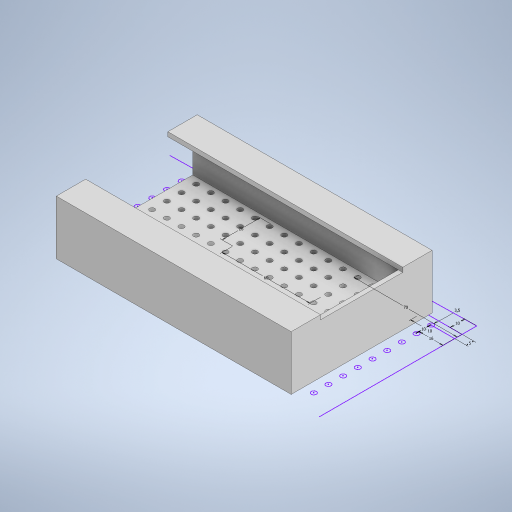
# Autodesk Inventor part: support batterie
Saved by Autodesk Inventor 2024 (Build 280153000, 153)
## iProperties
Created: 2024-02-10
Part Number: support batterie
Material: Generic
Document SubType Name: Modeling
Designer: Pooo
Density: 1 g/cm^3
Appearance: Default
Author: Pooo
## iProperties of the stored document support batterie_3DPrint.ipt
Created: 2024-02-22
Part Number: support batterie_3DPrint
Material: Generic
Document SubType Name: Modeling
Designer: Pooo
Density: 1 g/cm^3
Appearance: Default
Author: Pooo
Autodesk Inventor part; units mm, degrees
ref_plane "YZ Plane" through (0, 0, 0) normal (1, 0, 0) x (0, 1, 0)
ref_plane "XZ Plane" through (0, 0, 0) normal (0, 1, 0) x (-1, 0, 0)
ref_plane "XY Plane" through (0, 0, 0) normal (0, 0, 1) x (1, 0, 0)
sketch "Sketch1" plane through (0, 0, 0) normal (0, 1, 0) x (-1, 0, 0)
  point P0 (0, 0)
sketch "Sketch2" plane through (0, 0, 0) normal (0, 1, 0) x (-1, 0, 0)
  line L0 (43.1586, 43.7586) -> (-113.8414, 43.7586)
  line L1 (-113.8414, 43.7586) -> (-113.8414, -46.2414)
  line L2 (-113.8414, -46.2414) -> (43.1586, -46.2414)
  line L3 (43.1586, -46.2414) -> (43.1586, 43.7586)
  line L4 (43.1586, -46.2414) -> (-113.8414, -46.2414)
  line L5 (-113.8414, -46.2414) -> (-113.8414, -49.2414)
  line L6 (-113.8414, -49.2414) -> (43.1586, -49.2414)
  line L7 (43.1586, -49.2414) -> (43.1586, -46.2414)
  line L8 (43.1586, 43.7586) -> (-113.8414, 43.7586)
  line L9 (-113.8414, 43.7586) -> (-113.8414, 46.7586)
  line L10 (-113.8414, 46.7586) -> (43.1586, 46.7586)
  line L11 (43.1586, 46.7586) -> (43.1586, 43.7586)
  line L12 (-113.8414, 46.7586) -> (-116.8414, 46.7586)
  line L13 (-116.8414, 46.7586) -> (-116.8414, -49.2414)
  line L14 (-116.8414, -49.2414) -> (-113.8414, -49.2414)
  line L15 (-113.8414, -49.2414) -> (-113.8414, 46.7586)
  point P0 (0, 0)
  dimension "d0" = 90
  dimension "d1" = 157
  dimension "d2" = 3
  dimension "d3" = 3
  dimension "d4" = 3
  constraints: 32 end point, 8 parallel, 4 horizontal, 4 perpendicular
  measures "d0" distance of L2.end L0.start
  measures "d1" distance of L1.end L2.end
  measures "d2" distance of L4.end L5.end
  measures "d3" distance of L8.end L9.end
  measures "d4" distance of L14.end L13.end
extrude "Extrusion1" add sketch "Sketch2" along normal blind 3
sketch "Sketch3" plane through (0, 3, 0) normal (0, 1, 0) x (1, 0, 0)
  line L0 (-43.1586, -46.7586) -> (116.8414, -46.7586) projected
  line L1 (116.8414, -46.7586) -> (116.8414, 49.2414) projected
  line L2 (-43.1586, -46.7586) -> (116.8414, -46.7586)
  line L3 (116.8414, -46.7586) -> (116.8414, -43.7586)
  line L4 (116.8414, -43.7586) -> (-43.1586, -43.7586)
  line L5 (-43.1586, -43.7586) -> (-43.1586, -46.7586)
  line L6 (116.8414, 49.2414) -> (-43.1586, 49.2414) projected
  line L7 (-43.1586, 49.2414) -> (116.8414, 49.2414)
  line L8 (116.8414, 49.2414) -> (116.8414, 46.2414)
  line L9 (116.8414, 46.2414) -> (-43.1586, 46.2414)
  line L10 (-43.1586, 46.2414) -> (-43.1586, 49.2414)
  line L11 (116.8414, -43.7586) -> (113.8414, -43.7586)
  line L12 (113.8414, -43.7586) -> (113.8414, 46.2414)
  line L13 (113.8414, 46.2414) -> (116.8414, 46.2414)
  line L14 (116.8414, 46.2414) -> (116.8414, -43.7586)
  point P0 (0, 0)
  dimension "d7" = 3
  dimension "d8" = 3
  dimension "d9" = 3
  constraints: 24 end point, 6 parallel, 3 horizontal, 3 perpendicular, 3 point on line
  measures "d7" distance of L3.end L2.end
  measures "d8" distance of L7.end L8.end
  measures "d9" distance of L12.end L13.end
extrude "Extrusion3" add sketch "Sketch3" along normal blind 31
sketch "Sketch8" plane through (0, 34, 0) normal (0, 1, 0) x (1, 0, 0)
  line L0 (116.8414, -46.7586) -> (116.8414, 49.2414) projected
  line L1 (-43.1586, 49.2414) -> (116.8414, 49.2414)
  line L2 (116.8414, 49.2414) -> (116.8414, 29.2414)
  line L3 (116.8414, 29.2414) -> (-43.1586, 29.2414)
  line L4 (-43.1586, 29.2414) -> (-43.1586, 49.2414)
  line L5 (116.8414, -46.7586) -> (-43.1586, -46.7586)
  line L6 (-43.1586, -46.7586) -> (-43.1586, -26.7586)
  line L7 (-43.1586, -26.7586) -> (116.8414, -26.7586)
  line L8 (116.8414, -26.7586) -> (116.8414, -46.7586)
  point P0 (0, 0)
  dimension "d23" = 20
  dimension "d24" = 20
  constraints: 16 end point, 4 parallel, 2 horizontal, 2 perpendicular, 2 point on line
  measures "d23" distance of L1.end L2.end
  measures "d24" distance of L5.end L6.end
extrude "Extrusion4" add sketch "Sketch8" along normal blind 3
sketch "Sketch12" plane through (-65.6586, 0, -52.9186) normal (0, -1, 0) x (0, 0, -1)
  line L0 (0, 0) -> (3.9725, 205.1618)
  line L1 (3.9725, 205.1618) -> (-6.0275, 205.1618)
  line L2 (-103.3545, 205.1618) -> (3.9725, 205.1618)
  line L3 (-6.0275, 205.1618) -> (-11.0275, 205.1618)
  line L4 (-11.0275, 205.1618) -> (-11.0275, 189.1618)
  circle A0 centre (-11.0275, 189.1618) radius 1.75
  circle A1 centre (-11.0275, 179.1618) radius 1.75
  circle A2 centre (-11.0275, 169.1618) radius 1.75
  circle A3 centre (-11.0275, 159.1618) radius 1.75
  circle A4 centre (-11.0275, 149.1618) radius 1.75
  circle A5 centre (-11.0275, 139.1618) radius 1.75
  circle A6 centre (-11.0275, 129.1618) radius 1.75
  circle A7 centre (-11.0275, 119.1618) radius 1.75
  circle A8 centre (-11.0275, 109.1618) radius 1.75
  circle A9 centre (-11.0275, 99.1618) radius 1.75
  circle A10 centre (-11.0275, 89.1618) radius 1.75
  circle A11 centre (-11.0275, 79.1618) radius 1.75
  circle A12 centre (-11.0275, 69.1618) radius 1.75
  circle A13 centre (-11.0275, 59.1618) radius 1.75
  circle A14 centre (-11.0275, 49.1618) radius 1.75
  circle A15 centre (-11.0275, 39.1618) radius 1.75
  circle A16 centre (-11.0275, 29.1618) radius 1.75
  circle A17 centre (-11.0275, 19.1618) radius 1.75
  circle A18 centre (-21.0275, 189.1618) radius 1.75
  circle A19 centre (-21.0275, 179.1618) radius 1.75
  circle A20 centre (-21.0275, 169.1618) radius 1.75
  circle A21 centre (-21.0275, 159.1618) radius 1.75
  circle A22 centre (-21.0275, 149.1618) radius 1.75
  circle A23 centre (-21.0275, 139.1618) radius 1.75
  circle A24 centre (-21.0275, 129.1618) radius 1.75
  circle A25 centre (-21.0275, 119.1618) radius 1.75
  circle A26 centre (-21.0275, 109.1618) radius 1.75
  circle A27 centre (-21.0275, 99.1618) radius 1.75
  circle A28 centre (-21.0275, 89.1618) radius 1.75
  circle A29 centre (-21.0275, 79.1618) radius 1.75
  circle A30 centre (-21.0275, 69.1618) radius 1.75
  circle A31 centre (-21.0275, 59.1618) radius 1.75
  circle A32 centre (-21.0275, 49.1618) radius 1.75
  circle A33 centre (-21.0275, 39.1618) radius 1.75
  circle A34 centre (-21.0275, 29.1618) radius 1.75
  circle A35 centre (-21.0275, 19.1618) radius 1.75
  circle A36 centre (-31.0275, 189.1618) radius 1.75
  circle A37 centre (-31.0275, 179.1618) radius 1.75
  circle A38 centre (-31.0275, 169.1618) radius 1.75
  circle A39 centre (-31.0275, 159.1618) radius 1.75
  circle A40 centre (-31.0275, 149.1618) radius 1.75
  circle A41 centre (-31.0275, 139.1618) radius 1.75
  circle A42 centre (-31.0275, 129.1618) radius 1.75
  circle A43 centre (-31.0275, 119.1618) radius 1.75
  circle A44 centre (-31.0275, 109.1618) radius 1.75
  circle A45 centre (-31.0275, 99.1618) radius 1.75
  circle A46 centre (-31.0275, 89.1618) radius 1.75
  circle A47 centre (-31.0275, 79.1618) radius 1.75
  circle A48 centre (-31.0275, 69.1618) radius 1.75
  circle A49 centre (-31.0275, 59.1618) radius 1.75
  circle A50 centre (-31.0275, 49.1618) radius 1.75
  circle A51 centre (-31.0275, 39.1618) radius 1.75
  circle A52 centre (-31.0275, 29.1618) radius 1.75
  circle A53 centre (-31.0275, 19.1618) radius 1.75
  circle A54 centre (-41.0275, 189.1618) radius 1.75
  circle A55 centre (-41.0275, 179.1618) radius 1.75
  circle A56 centre (-41.0275, 169.1618) radius 1.75
  circle A57 centre (-41.0275, 159.1618) radius 1.75
  circle A58 centre (-41.0275, 149.1618) radius 1.75
  circle A59 centre (-41.0275, 139.1618) radius 1.75
  circle A60 centre (-41.0275, 129.1618) radius 1.75
  circle A61 centre (-41.0275, 119.1618) radius 1.75
  circle A62 centre (-41.0275, 109.1618) radius 1.75
  circle A63 centre (-41.0275, 99.1618) radius 1.75
  circle A64 centre (-41.0275, 89.1618) radius 1.75
  circle A65 centre (-41.0275, 79.1618) radius 1.75
  circle A66 centre (-41.0275, 69.1618) radius 1.75
  circle A67 centre (-41.0275, 59.1618) radius 1.75
  circle A68 centre (-41.0275, 49.1618) radius 1.75
  circle A69 centre (-41.0275, 39.1618) radius 1.75
  circle A70 centre (-41.0275, 29.1618) radius 1.75
  circle A71 centre (-41.0275, 19.1618) radius 1.75
  circle A72 centre (-51.0275, 189.1618) radius 1.75
  circle A73 centre (-51.0275, 179.1618) radius 1.75
  circle A74 centre (-51.0275, 169.1618) radius 1.75
  circle A75 centre (-51.0275, 159.1618) radius 1.75
  circle A76 centre (-51.0275, 149.1618) radius 1.75
  circle A77 centre (-51.0275, 139.1618) radius 1.75
  circle A78 centre (-51.0275, 129.1618) radius 1.75
  circle A79 centre (-51.0275, 119.1618) radius 1.75
  circle A80 centre (-51.0275, 109.1618) radius 1.75
  circle A81 centre (-51.0275, 99.1618) radius 1.75
  circle A82 centre (-51.0275, 89.1618) radius 1.75
  circle A83 centre (-51.0275, 79.1618) radius 1.75
  circle A84 centre (-51.0275, 69.1618) radius 1.75
  circle A85 centre (-51.0275, 59.1618) radius 1.75
  circle A86 centre (-51.0275, 49.1618) radius 1.75
  circle A87 centre (-51.0275, 39.1618) radius 1.75
  circle A88 centre (-51.0275, 29.1618) radius 1.75
  circle A89 centre (-51.0275, 19.1618) radius 1.75
  circle A90 centre (-61.0275, 189.1618) radius 1.75
  circle A91 centre (-61.0275, 179.1618) radius 1.75
  circle A92 centre (-61.0275, 169.1618) radius 1.75
  circle A93 centre (-61.0275, 159.1618) radius 1.75
  circle A94 centre (-61.0275, 149.1618) radius 1.75
  circle A95 centre (-61.0275, 139.1618) radius 1.75
  circle A96 centre (-61.0275, 129.1618) radius 1.75
  circle A97 centre (-61.0275, 119.1618) radius 1.75
  circle A98 centre (-61.0275, 109.1618) radius 1.75
  circle A99 centre (-61.0275, 99.1618) radius 1.75
  circle A100 centre (-61.0275, 89.1618) radius 1.75
  circle A101 centre (-61.0275, 79.1618) radius 1.75
  circle A102 centre (-61.0275, 69.1618) radius 1.75
  circle A103 centre (-61.0275, 59.1618) radius 1.75
  circle A104 centre (-61.0275, 49.1618) radius 1.75
  circle A105 centre (-61.0275, 39.1618) radius 1.75
  circle A106 centre (-61.0275, 29.1618) radius 1.75
  circle A107 centre (-61.0275, 19.1618) radius 1.75
  circle A108 centre (-71.0275, 189.1618) radius 1.75
  circle A109 centre (-71.0275, 179.1618) radius 1.75
  circle A110 centre (-71.0275, 169.1618) radius 1.75
  circle A111 centre (-71.0275, 159.1618) radius 1.75
  circle A112 centre (-71.0275, 149.1618) radius 1.75
  circle A113 centre (-71.0275, 139.1618) radius 1.75
  circle A114 centre (-71.0275, 129.1618) radius 1.75
  circle A115 centre (-71.0275, 119.1618) radius 1.75
  circle A116 centre (-71.0275, 109.1618) radius 1.75
  circle A117 centre (-71.0275, 99.1618) radius 1.75
  circle A118 centre (-71.0275, 89.1618) radius 1.75
  circle A119 centre (-71.0275, 79.1618) radius 1.75
  circle A120 centre (-71.0275, 69.1618) radius 1.75
  circle A121 centre (-71.0275, 59.1618) radius 1.75
  circle A122 centre (-71.0275, 49.1618) radius 1.75
  circle A123 centre (-71.0275, 39.1618) radius 1.75
  circle A124 centre (-71.0275, 29.1618) radius 1.75
  circle A125 centre (-71.0275, 19.1618) radius 1.75
  circle A126 centre (-81.0275, 189.1618) radius 1.75
  circle A127 centre (-81.0275, 179.1618) radius 1.75
  circle A128 centre (-81.0275, 169.1618) radius 1.75
  circle A129 centre (-81.0275, 159.1618) radius 1.75
  circle A130 centre (-81.0275, 149.1618) radius 1.75
  circle A131 centre (-81.0275, 139.1618) radius 1.75
  circle A132 centre (-81.0275, 129.1618) radius 1.75
  circle A133 centre (-81.0275, 119.1618) radius 1.75
  circle A134 centre (-81.0275, 109.1618) radius 1.75
  circle A135 centre (-81.0275, 99.1618) radius 1.75
  circle A136 centre (-81.0275, 89.1618) radius 1.75
  circle A137 centre (-81.0275, 79.1618) radius 1.75
  circle A138 centre (-81.0275, 69.1618) radius 1.75
  circle A139 centre (-81.0275, 59.1618) radius 1.75
  circle A140 centre (-81.0275, 49.1618) radius 1.75
  circle A141 centre (-81.0275, 39.1618) radius 1.75
  circle A142 centre (-81.0275, 29.1618) radius 1.75
  circle A143 centre (-81.0275, 19.1618) radius 1.75
  circle A144 centre (-91.0275, 189.1618) radius 1.75
  circle A145 centre (-91.0275, 179.1618) radius 1.75
  circle A146 centre (-91.0275, 169.1618) radius 1.75
  circle A147 centre (-91.0275, 159.1618) radius 1.75
  circle A148 centre (-91.0275, 149.1618) radius 1.75
  circle A149 centre (-91.0275, 139.1618) radius 1.75
  circle A150 centre (-91.0275, 129.1618) radius 1.75
  circle A151 centre (-91.0275, 119.1618) radius 1.75
  circle A152 centre (-91.0275, 109.1618) radius 1.75
  circle A153 centre (-91.0275, 99.1618) radius 1.75
  circle A154 centre (-91.0275, 89.1618) radius 1.75
  circle A155 centre (-91.0275, 79.1618) radius 1.75
  circle A156 centre (-91.0275, 69.1618) radius 1.75
  circle A157 centre (-91.0275, 59.1618) radius 1.75
  circle A158 centre (-91.0275, 49.1618) radius 1.75
  circle A159 centre (-91.0275, 39.1618) radius 1.75
  circle A160 centre (-91.0275, 29.1618) radius 1.75
  circle A161 centre (-91.0275, 19.1618) radius 1.75
  line L5 (-6.0275, 205.1618) -> (-6.0275, 135.1618)
  point P0 (-54.6545, 5)
  point P1 (-32.0275, 75.1618)
  point P2 (-32.0275, 135.1618)
  point P3 (-6.0275, 75.1618)
  dimension "d59" = 10
  dimension "d58" = 5
  dimension "d57" = 16
  dimension "d56" = 3.5
  dimension "d47" = 10
  dimension "d46" = 10
  dimension "d55" = 70
  dimension "d53" = 26
  dimension "d54" = 60
  constraints: 162 centre point, 12 end point, 2 point on line, 2 vertical, 1 coincident, 1 horizontal, 1 perpendicular, 322 other
  measures "d59" distance of L0.end L1.end
  measures "d58" distance of L1.end L3.end
  measures "d57" distance of L3.end L4.end
  measures "d56" diameter of A0
  measures "d47" distance of A0.centre A1.centre
  measures "d46" distance of A0.centre A18.centre
  measures "d55" distance of L1.end L5.end
  measures "d53" distance of point (-6.027, 75.162) point (-32.027, 75.162)
  measures "d54" distance of point (-32.027, 75.162) point (-32.027, 135.162)
extrude "Extrusion7" cut sketch "Sketch12" against normal blind 20 contours A2 | A3 | A4 | A5 | A6 | A7 | A8 | A9 | A10 | A11 | A12 | A13 | A14 | A15 | A16 | A20 | A21 | A22 | A23 | A24 | A25 | A26 | A27 | A28 | A29 | A30 | A31 | A32 | A33 | A34 | A38 | A39 | A40 | A41 | A42 | A43 | A44 | A45 | A46 | A47 | A48 | A49 | A50 | A51 | A52 | A56 | A57 | A58 | A59 | A60 | A61 | A62 | A63 | A64 | A65 | A66 | A67 | A68 | A69 | A70 | A74 | A75 | A76 | A77 | A78 | A79 | A80 | A81 | A82 | A83 | A84 | A85 | A86 | A87 | A88 | A92 | A93 | A94 | A95 | A96 | A97 | A98 | A99 | A100 | A101 | A102 | A103 | A104 | A105 | A106 | A110 | A111 | A112 | A113 | A114 | A115 | A116 | A117 | A118 | A119 | A120 | A121 | A122 | A123 | A124 | A128 | A129 | A130 | A131 | A132 | A133 | A134 | A135 | A136 | A137 | A138 | A139 | A140 | A141 | A142 | A146 | A147 | A148 | A149 | A150 | A151 | A152 | A153 | A154 | A155 | A156 | A157 | A158 | A159 | A160
body "Solid1"
